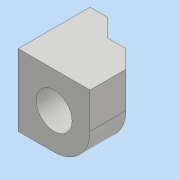
# Autodesk Inventor part: 20
Saved by Autodesk Inventor 2017 (Build 210142000, 142)
## iProperties
Part Number: 20
Material: 一般
Document SubType Name: Modeling
Designer: d8910
Density: 1 g/cm^3
Appearance: 預設
Author: d8910
Autodesk Inventor part; units mm, degrees
ref_plane "YZ Plane" through (0, 0, 0) normal (1, 0, 0) x (0, 1, 0)
ref_plane "XZ Plane" through (0, 0, 0) normal (0, 1, 0) x (-1, 0, 0)
ref_plane "XY Plane" through (0, 0, 0) normal (0, 0, 1) x (1, 0, 0)
sketch "草圖2" plane through (0, 0, 0) normal (0, 1, 0) x (-1, 0, 0)
  line L0 (10, 10) -> (-10, 10)
  line L1 (-10, 10) -> (-10, 0)
  line L2 (-10, -10) -> (0, -10) construction
  line L3 (10, -10) -> (10, 10)
  arc A0 (-10, 0) -> (0, -10) centre (0, 0) ccw
  line L4 (-10, 0) -> (-10, -10) construction
  line L5 (0, -10) -> (10, -10)
  circle A1 centre (0, 0) radius 5
  point P0 (0, 0)
  point P1 (10, 0)
  dimension "d2" = 20
  dimension "d3" = 20
  dimension "d4" = 10
  dimension "d5" = 10
  dimension "d6" = 10
  constraints: 12 end point, 4 parallel, 2 centre point, 2 perpendicular, 2 point on circle, 2 tangent, 1 coincident, 1 horizontal, 1 horizontal alignment, 1 midpoint, 1 vertical alignment
  measures "d2" distance of L3.start L0.start
  measures "d3" distance of L2.start L3.start
  measures "d4" radius of A0
  measures "d5" distance from line of L1 point (0, 0)
  measures "d6" diameter of A1
extrude "擠出1" add sketch "草圖2" along normal blind 10
sketch "草圖3" plane through (-10, 0, 10) normal (0, 0, 1) x (1, 0, 0)
  line L0 (0, 10) -> (20, 10) projected
  line L1 (20, 10) -> (15, 15)
  line L2 (15, 15) -> (10, 15)
  line L3 (10, 15) -> (5, 20)
  line L4 (5, 20) -> (0, 20)
  line L5 (0, 20) -> (0, 10)
  point P0 (10, 0)
  dimension "d9" = 5
  dimension "d10" = 5
  dimension "d11" = 5
  dimension "d12" = 5
  dimension "d13" = 10
  constraints: 10 end point, 2 parallel, 1 perpendicular
  measures "d9" distance of L3.end L4.end
  measures "d10" horizontal distance of L3.end L2.end
  measures "d11" distance of L1.end L2.end
  measures "d12" distance from line of L0 L1.end
  measures "d13" distance between parallel lines of L0 L4
extrude "擠出2" add sketch "草圖3" against normal blind 5
sketch "草圖4" plane through (-10, 0, -10) normal (-1, 0, 0) x (0, 0, 1)
  line L0 (15, 10) -> (15, 20) projected
  line L1 (15, 20) -> (10, 15)
  line L2 (10, 15) -> (10, 10)
  line L3 (10, 0) -> (10, 10) projected
  line L4 (15, 10) -> (10, 10)
  dimension "d16" = 5
  dimension "d17" = 5
  constraints: 6 end point, 1 collinear, 1 horizontal
  measures "d16" horizontal distance of L1.end L0.end
  measures "d17" distance between parallel lines of L0 L2
extrude "擠出3" add sketch "草圖4" against normal blind 5
sketch "草圖5" plane through (0, 10, 0) normal (0, 1, 0) x (1, 0, 0)
  line L0 (-10, 10) -> (-5, 10)
  line L1 (-5, 10) -> (-5, 5)
  line L2 (-5, 5) -> (-10, 5)
  line L3 (-10, 5) -> (-10, 10)
  line L4 (-5, 0) -> (-5, -5) projected
  point P0 (0, 0)
  dimension "d20" = 5
  dimension "d21" = 5
  constraints: 8 end point, 3 equal length, 1 horizontal, 1 perpendicular
  measures "d20" distance of L1.end L2.end
  measures "d21" distance of L2.end L0.start
extrude "擠出4" add sketch "草圖5" along normal blind 5
